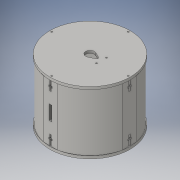
# Autodesk Inventor part: Cyldr_Motor
Saved by Autodesk Inventor 2016 (Build 200138000, 138)
## iProperties
Created: 2019-03-07
Part Number: Cyldr_Motor
Material: Generic
Document SubType Name: Modeling
Designer: student
Density: 1 g/cm^3
Appearance: Default
Author: student
Autodesk Inventor part; units mm, degrees
ref_plane "YZ Plane" through (0, 0, 0) normal (1, 0, 0) x (0, 1, 0)
ref_plane "XZ Plane" through (0, 0, 0) normal (0, 1, 0) x (-1, 0, 0)
ref_plane "XY Plane" through (0, 0, 0) normal (0, 0, 1) x (1, 0, 0)
sketch "Sketch1" plane through (0, 0, 0) normal (0, 1, 0) x (-1, 0, 0)
  circle A0 centre (0, 0) radius 70.993
  circle A1 centre (0, 0) radius 6.35 construction
  line L0 (0, 6.35) -> (-19.05, 6.35) construction
  circle A2 centre (-11.684, 0) radius 1.905 construction
  line L1 (-11.684, 0) -> (-19.05, 0) construction
  line L2 (-19.05, 0) -> (-20.3962, 0) construction
  line L3 (-20.3962, 0) -> (-20.3962, 7.4295) construction
  line L4 (-20.3962, 0) -> (-20.3962, -7.4295) construction
  line L5 (-20.3962, 7.4295) -> (-20.3962, 8.7757) construction
  circle A3 centre (-20.3962, 8.7757) radius 1.3462
  line L6 (-20.3962, -7.4295) -> (-20.3962, -8.7757) construction
  circle A4 centre (-20.3962, -8.7757) radius 1.3462
  arc A5 (-3.3157, -6.8608) -> (-3.3157, 6.8608) centre (0, 0) ccw
  arc A6 (-12.6572, 2.3462) -> (-12.6572, -2.3462) centre (-11.684, 0) ccw
  line L7 (-12.6572, 2.3462) -> (-3.3157, 6.8608)
  line L8 (-12.6572, -2.3462) -> (-3.3157, -6.8608)
  dimension "d1" = 12.7
  dimension "d0" = 141.986
  dimension "d2" = 19.05
  dimension "d3" = 3.429
  dimension "d4" = 3.81
  dimension "d5" = 1.3462
  dimension "d6" = 7.4295
  dimension "d7" = 7.4295
  dimension "d8" = 1.3462
  dimension "d9" = 1.3462
  dimension "d10" = 15.24
  dimension "d11" = 5.08
  dimension "d13" = 20.3962
  dimension "d14" = 51.588
  dimension "d15" = 7.8102
  dimension "d16" = 9.1564
  dimension "d17" = 0.6309
  dimension "d92" = 63.373
  constraints: 18 end point, 5 coincident, 4 centre point, 4 horizontal, 4 point on circle, 4 vertical, 3 vertical alignment, 2 tangent, 6 other
  measures "d0" diameter of A0
  measures "d2" distance of L0.start L0.end
  measures "d4" diameter of A2
  measures "d5" distance of L1.end L2.end
  measures "d6" distance of L2.end L3.end
  measures "d7" distance of L2.end L4.end
  measures "d8" distance of L3.end L5.end
  measures "d9" distance of L4.end L6.end
  measures "d10" diameter of A5
  measures "d11" diameter of A6
  measures "d13" horizontal distance of A0.centre point (-20.396, 8.776)
  measures "d14" angle of L8 L7
  measures "d16" distance from line of point (-20.396, -8.776) L8
  measures "d17" distance edge to line of A2 L8
  measures "d92" radial gap between concentric circles of A0 A5
extrude "Extrusion1" add sketch "Sketch1" along normal blind 4.572
sketch "Sketch2" plane through (0, 0, 0) normal (0, -1, 0) x (1, 0, 0)
  arc A0 (3.3157, 6.8608) -> (3.3157, -6.8608) centre (0, 0) ccw projected
  circle A1 centre (0, 0) radius 69.85 construction
  circle A2 centre (0, 0) radius 65.278
  line L0 (-69.85, 0) -> (-57.15, 0) construction
  line L1 (-69.85, 0) -> (-57.15, 0) construction
  line L2 (0, 69.85) -> (12.7, 69.85) construction
  line L3 (69.85, 0) -> (82.55, 0) construction
  line L4 (69.85, 0) -> (82.55, 0) construction
  line L5 (12.7, -69.85) -> (69.85, -12.7) construction
  line L6 (41.275, -41.275) -> (59.2355, -59.2355) construction
  line L7 (41.275, -41.275) -> (66.675, -41.275) construction
  arc A3 (12.7, -69.85) -> (69.85, -12.7) centre (-4.968, 4.968) ccw
  line L8 (-12.7, -69.85) -> (-69.85, -12.7) construction
  line L9 (-41.275, -41.275) -> (-59.2355, -59.2355) construction
  line L10 (-41.275, -41.275) -> (-15.875, -41.275) construction
  arc A4 (-69.85, -12.7) -> (-12.7, -69.85) centre (4.968, 4.968) ccw
  line L11 (-69.85, 12.7) -> (-12.7, 69.85) construction
  line L12 (12.7, 69.85) -> (69.85, 12.7) construction
  line L13 (-41.275, 41.275) -> (-59.2355, 59.2355) construction
  line L14 (41.275, 41.275) -> (59.2355, 59.2355) construction
  arc A5 (-12.7, 69.85) -> (-69.85, 12.7) centre (4.968, -4.968) ccw
  arc A6 (69.85, 12.7) -> (12.7, 69.85) centre (-4.968, -4.968) ccw
  line L15 (-69.85, -12.7) -> (-69.85, 12.7)
  line L16 (-12.7, 69.85) -> (12.7, 69.85)
  line L17 (69.85, 12.7) -> (69.85, -12.7)
  line L18 (-12.7, -69.85) -> (12.7, -69.85)
  dimension "d20" = 139.7
  dimension "d21" = 130.556
  dimension "d47" = 12.7
  dimension "d49" = 12.7
  dimension "d53" = 12.7
  dimension "d58" = 12.7
  dimension "d60" = 12.7
  dimension "d62" = 25.4
  dimension "d63" = 45
  dimension "d64" = 25.4
  dimension "d65" = 135
  dimension "d66" = 25.4
  dimension "d67" = 90
  dimension "d68" = 25.4
  dimension "d69" = 90
  dimension "d70" = 76.8758
  dimension "d71" = 76.8758
  dimension "d72" = 76.8758
  dimension "d73" = 76.8758
  dimension "d74" = 4.968
  dimension "d75" = 25.4
  dimension "d76" = 74.818
  dimension "d77" = 25.4
  dimension "d78" = 74.818
  dimension "d79" = 25.4
  dimension "d80" = 74.818
  dimension "d81" = 74.818
  dimension "d82" = 25.4
  dimension "d83" = 74.818
  dimension "d84" = 74.818
  constraints: 38 end point, 11 point on circle, 8 horizontal, 6 centre point, 4 midpoint, 2 coincident, 2 equal length, 2 vertical, 1 collinear
  measures "d20" diameter of A1
  measures "d21" diameter of A2
  measures "d47" distance of L0.start L11.start
  measures "d49" distance of L0.start L8.end
  measures "d53" distance of L2.start L11.end
  measures "d58" distance of L3.start L12.end
  measures "d60" distance of L3.start L5.end
  measures "d62" distance of L6.start L6.end
  measures "d63" angle of L6 L7
  measures "d64" distance of L9.start L9.end
  measures "d65" angle of L9 L10
  measures "d66" distance of L13.start L13.end
  measures "d67" angle of L11 L13
  measures "d68" distance of L14.start L14.end
  measures "d69" angle of L14 L12
  measures "d70" radius of A6
  measures "d71" radius of A3
  measures "d72" radius of A4
  measures "d73" radius of A5
  measures "d74" horizontal distance of A5.centre A0.centre
  measures "d75" distance of L8.end L15.end
  measures "d76" distance from line of A5.centre L15
  measures "d77" distance of L11.end L2.end
  measures "d78" distance from line of A5.centre L16
  measures "d79" distance of L12.end L17.end
  measures "d80" distance from line of A6.centre L17
  measures "d81" distance from line of A3.centre L17
  measures "d82" distance of L8.start L5.start
  measures "d83" distance from line of L18 A4.centre
  measures "d84" distance from line of A3.centre L18
extrude "Extrusion7" add sketch "Sketch2" along normal blind 101.6
sketch "Sketch4" plane through (0, 0, 0) normal (1, 0, 0) x (0, 1, 0)
  line L0 (0, 1.3335) -> (0, -1.3335)
  line L1 (-17.78, -1.3335) -> (-17.78, 1.3335)
  line L2 (-11.9594, -2.921) -> (-9.2924, -2.921)
  line L3 (-9.2924, 2.921) -> (-11.9594, 2.921)
  line L4 (-9.2924, -2.921) -> (-9.2924, -1.3335)
  line L5 (-9.2924, 1.3335) -> (-9.2924, 2.921)
  line L6 (-17.78, 1.3335) -> (-11.9594, 1.3335)
  line L7 (-9.2924, 1.3335) -> (0, 1.3335)
  line L8 (0, -1.3335) -> (-9.2924, -1.3335)
  line L9 (-11.9594, -1.3335) -> (-17.78, -1.3335)
  line L10 (-11.9594, 2.921) -> (-11.9594, 1.3335)
  line L11 (-11.9594, -1.3335) -> (-11.9594, -2.921)
  line L12 (0, 65.278) -> (-101.6, 65.278) projected
  line L13 (-50.8, 65.278) -> (-50.8, -65.278)
  line L14 (0, -65.278) -> (-101.6, -65.278) projected
  line L15 (-101.6, 1.3335) -> (-101.6, -1.3335)
  line L16 (-83.82, -1.3335) -> (-83.82, 1.3335)
  line L17 (-89.6406, -2.921) -> (-92.3076, -2.921)
  line L18 (-92.3076, 2.921) -> (-89.6406, 2.921)
  line L19 (-92.3076, -2.921) -> (-92.3076, -1.3335)
  line L20 (-92.3076, 1.3335) -> (-92.3076, 2.921)
  line L21 (-83.82, 1.3335) -> (-89.6406, 1.3335)
  line L22 (-92.3076, 1.3335) -> (-101.6, 1.3335)
  line L23 (-101.6, -1.3335) -> (-92.3076, -1.3335)
  line L24 (-89.6406, -1.3335) -> (-83.82, -1.3335)
  line L25 (-89.6406, 2.921) -> (-89.6406, 1.3335)
  line L26 (-89.6406, -1.3335) -> (-89.6406, -2.921)
  point P0 (0, 0)
  point P1 (-101.6, 0)
  dimension "d29" = 2.667
  dimension "d30" = 5.842
  dimension "d31" = 2.667
  dimension "d32" = 5.842
  dimension "d33" = 1.5875
  dimension "d34" = 1.5875
  dimension "d35" = 1.5875
  dimension "d36" = 5.8206
  dimension "d37" = 2.667
  dimension "d38" = 17.78
  dimension "d41" = 62.357
  dimension "d42" = 33.02
  constraints: 50 end point, 13 symmetric about line, 10 parallel, 4 perpendicular, 3 horizontal, 2 midpoint
  measures "d29" distance of L3.end L3.start
  measures "d30" distance of L3.start L2.end
  measures "d31" distance between parallel lines of L7 L8
  measures "d32" distance between parallel lines of L2 L3
  measures "d33" distance of L5.start L3.start
  measures "d34" distance of L3.end L6.end
  measures "d35" distance of L9.start L2.start
  measures "d36" distance of L1.end L6.end
  measures "d37" distance of L2.start L2.end
  measures "d38" distance between parallel lines of L1 L0
  measures "d41" distance between parallel lines of L12 L3
  measures "d42" distance between parallel lines of L13 L1
extrude "Extrusion8" cut sketch "Sketch4" along normal mid plane 254
sketch "Sketch6" plane through (0, -101.6, 0) normal (0, -1, 0) x (1, 0, 0)
  arc A0 (-69.85, -12.7) -> (-12.7, -69.85) centre (4.968, 4.968) ccw projected
  circle A1 centre (0, 0) radius 70.9952
  dimension "d91" = 141.9903
  constraints: 1 coincident, 3 other
extrude "Extrusion9" add sketch "Sketch6" along normal blind 4.572
sketch "Sketch7" plane through (-12.6879, 0, 69.85) normal (0, 0, 1) x (1, 0, 0)
  line L0 (11.3544, -17.78) -> (14.0214, -17.78)
  line L1 (11.3544, -11.9634) -> (9.7542, -11.9634)
  line L2 (9.7542, -11.9634) -> (9.7542, -9.2964)
  line L3 (9.7542, -9.2964) -> (11.3544, -9.2964)
  line L4 (11.3544, -17.78) -> (11.3544, -11.9634)
  line L5 (11.3544, -9.2964) -> (11.3544, 0)
  line L6 (14.0214, -9.2964) -> (15.6216, -9.2964)
  line L7 (14.0214, -11.9634) -> (15.6216, -11.9634)
  line L8 (15.6216, -11.9634) -> (15.6216, -9.2964)
  line L9 (14.0214, -17.78) -> (14.0214, -11.9634)
  line L10 (14.0214, -9.2964) -> (14.0214, 0)
  line L11 (-0.0121, -50.8) -> (25.3759, -50.8)
  line L12 (11.3544, -83.82) -> (14.0214, -83.82)
  line L13 (11.3544, -89.6366) -> (9.7542, -89.6366)
  line L14 (9.7542, -89.6366) -> (9.7542, -92.3036)
  line L15 (9.7542, -92.3036) -> (11.3544, -92.3036)
  line L16 (11.3544, -83.82) -> (11.3544, -89.6366)
  line L17 (11.3544, -92.3036) -> (11.3544, -101.6)
  line L18 (14.0214, -92.3036) -> (15.6216, -92.3036)
  line L19 (14.0214, -89.6366) -> (15.6216, -89.6366)
  line L20 (15.6216, -89.6366) -> (15.6216, -92.3036)
  line L21 (14.0214, -83.82) -> (14.0214, -89.6366)
  line L22 (14.0214, -92.3036) -> (14.0214, -101.6)
  line L23 (11.3544, 0) -> (14.0214, 0)
  line L24 (11.3544, -101.6) -> (14.0214, -101.6)
  point P0 (12.6879, 0)
  dimension "d106" = 1.6002
  dimension "d107" = 2.667
  dimension "d108" = 1.6002
  dimension "d109" = 9.2964
  dimension "d110" = 9.2964
  dimension "d111" = 1.6002
  dimension "d112" = 2.667
  dimension "d113" = 5.8166
  dimension "d114" = 2.667
  constraints: 50 end point, 12 symmetric about line, 5 horizontal, 4 parallel, 3 perpendicular, 3 vertical
  measures "d106" distance of L1.start L1.end
  measures "d107" distance of L1.end L2.end
  measures "d108" distance of L6.start L6.end
  measures "d109" distance of L3.end L5.end
  measures "d110" distance of L6.start L10.end
  measures "d111" distance of L7.start L7.end
  measures "d112" distance of L7.end L6.end
  measures "d113" distance of L0.end L7.start
  measures "d114" distance of L0.start L0.end
extrude "Extrusion10" cut sketch "Sketch7" against normal blind 254
sketch "Sketch8" plane through (0, 4.572, 0) normal (0, 1, 0) x (1, 0, 0)
  circle A0 centre (0, -67.5572) radius 1.3335
  line L0 (-1.3335, -69.85) -> (-1.3335, -65.2644) projected
  circle A1 centre (-67.5572, 0) radius 1.3335
  circle A2 centre (0, 67.5572) radius 1.3335
  circle A3 centre (67.5572, 0) radius 1.3335
  point P0 (0, 0)
  constraints: 4 centre point, 1 tangent
extrude "Extrusion11" cut sketch "Sketch8" against normal blind 5.08
sketch "Sketch9" plane through (0, -106.172, 0) normal (0, -1, 0) x (1, 0, 0)
  arc A0 (-67.5572, 1.3335) -> (-67.5572, -1.3335) centre (-67.5572, 0) ccw projected
  circle A1 centre (-67.5572, 0) radius 1.3335
  arc A2 (-1.3335, 67.5572) -> (1.3335, 67.5572) centre (0, 67.5572) ccw projected
  circle A3 centre (0, 67.5572) radius 1.3335
  circle A4 centre (67.5572, 0) radius 1.3335 projected
  circle A5 centre (67.5572, 0) radius 1.3335
  circle A6 centre (0, -67.5572) radius 1.3335 projected
  circle A7 centre (0, -67.5572) radius 1.3335
  point P0 (0, 0)
  constraints: 4 centre point, 4 coincident
extrude "Extrusion12" cut sketch "Sketch9" against normal blind 5.08
sketch "Sketch10" plane through (-12.7, -101.6, 69.85) normal (0, 0, 1) x (1, 0, 0)
  line L0 (0, 0) -> (11.3665, 0) projected
  line L1 (0, 101.6) -> (0, 0) projected
  line L2 (0, 0) -> (0, 101.6)
  line L3 (0, 50.8) -> (12.7, 50.8)
  line L4 (15.113, 38.1) -> (10.287, 38.1)
  line L5 (10.287, 38.1) -> (10.287, 63.5)
  line L6 (10.287, 63.5) -> (15.113, 63.5)
  line L7 (15.113, 63.5) -> (15.113, 38.1)
  line L8 (15.113, 38.1) -> (10.287, 63.5) construction
  line L9 (10.287, 38.1) -> (15.113, 63.5) construction
  point P0 (12.7, 101.6)
  dimension "d125" = 4.826
  dimension "d126" = 25.4
  constraints: 16 end point, 3 equal length, 3 midpoint, 2 horizontal, 1 perpendicular
  measures "d125" distance of L5.end L6.end
  measures "d126" distance of L4.end L5.end
extrude "Extrusion13" cut sketch "Sketch10" against normal blind 5.08
body "Solid1"
